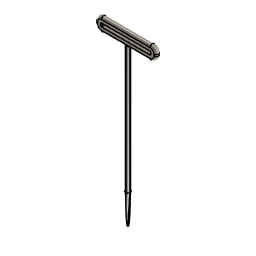
foamBrickElement (Autodesk Fusion 360 archive; units mm, degrees)
design "泡沫板_钉子"
Autodesk Fusion 360 part; units mm, degrees
sketch "草图1" plane through (0, 0, 0) normal (0, 1, 0) x (1, 0, 0)
  line L0 (0, 0) -> (0, -25.7)
  line L1 (0, -25.7) -> (-4.625, -25.7)
  line L2 (-4.625, -25.7) -> (-4.625, -28)
  line L3 (-4.625, -28) -> (5.375, -28)
  line L4 (5.375, -28) -> (5.375, -25.7)
  line L5 (5.375, -25.7) -> (0.75, -25.7)
  line L6 (0.75, -25.7) -> (0.75, 0)
  line L7 (0.75, 0) -> (0, 0)
  line L8 (0.375, -28) -> (0.375, 0)
  line L9 (0.375, 0) -> (0.375, -0.4348)
  line L10 (0.375, 0) -> (0.75, -5)
  line L11 (0.375, 0) -> (0, -5)
  line L12 (0.75, -5) -> (0, -5)
  dimension "d1" = 2.3
  dimension "d2" = 0.75
  dimension "d3" = 5
  dimension "d4" = 28
  dimension "d5" = 10
  constraint coincident L0.start L7.end
  constraint vertical L0
  constraint perpendicular L0 L1
  constraint perpendicular L1 L2
  constraint perpendicular L2 L3
  constraint perpendicular L2 L5
  constraint perpendicular L1 L6
  constraint perpendicular L0 L7
  constraint perpendicular L4 L5
  constraint midpoint L3 L8.start
  constraint midpoint L7 L8.end
  constraint perpendicular L3 L8
  constraint collinear L1 L5
  constraint coincident L8 L9.end
  constraint coincident L6 L10.end
  constraint coincident L0 L11.end
  constraint perpendicular L6 L12
  measures "d1" distance of L3.end L4.end
  measures "d2" distance of L0 L6
  measures "d3" distance of L7 L10.end
  measures "d4" distance of L3 L8.end
  measures "d5" distance of L2 L4
extrude "拉伸1" add sketch "草图1" along normal blind 0.75 contours L0 L1 L2 L3 L8 L12 | L8 L9 L11 L12 | L8 L9 L10 L12 | L3 L4 L5 L6 L8 L12
fillet "圆角1" radius 1 4 edges at (5.375, 0.375, 28) (5.375, 0.375, 25.7) (-4.625, 0.375, 25.7) (-4.625, 0.375, 28)
fillet "圆角2" radius 0.375 18 edges at (-1.8125, 0, 25.7) (-4.3321, 0, 25.9929) (-4.625, 0, 26.85) (-4.3321, 0, 27.7071) (0.375, 0, 28) (5.0821, 0, 27.7071) (5.375, 0, 26.85) (5.0821, 0, 25.9929) (2.5625, 0, 25.7) (-1.8125, 0.75, 25.7) (-4.3321, 0.75, 25.9929) (-4.625, 0.75, 26.85) (-4.3321, 0.75, 27.7071) (0.375, 0.75, 28) (5.0821, 0.75, 27.7071) (5.375, 0.75, 26.85) (5.0821, 0.75, 25.9929) (2.5625, 0.75, 25.7)
fillet "圆角3" radius 0.325 8 edges at (0.75, 0, 15.5375) (0.75, 0.75, 15.5375) (0, 0.75, 15.5375) (0, 0, 15.5375) (0.5625, 0, 2.5) (0.5625, 0.75, 2.5) (0.1875, 0, 2.5) (0.1875, 0.75, 2.5)
sketch "草图2" plane through (0, 0, 0) normal (0, -1, 0) x (1, 0, 0)
  line L0 (0.425, 26.075) -> (4.375, 26.075)
  arc A0 (4.375, 26.075) -> (5, 26.7) centre (4.375, 26.7) ccw
  line L1 (5, 26.7) -> (5, 27)
  arc A1 (5, 27) -> (4.375, 27.625) centre (4.375, 27) ccw
  line L2 (4.375, 27.625) -> (-3.625, 27.625)
  arc A2 (-3.625, 27.625) -> (-4.25, 27) centre (-3.625, 27) ccw
  line L3 (-4.25, 27) -> (-4.25, 26.7)
  arc A3 (-4.25, 26.7) -> (-3.625, 26.075) centre (-3.625, 26.7) ccw
  line L4 (-3.625, 26.075) -> (0.325, 26.075)
  line L5 (0.325, 26.075) -> (0.325, 5.0122)
  line L6 (0.325, 5.0122) -> (0.375, 4.3455)
  line L7 (0.375, 4.3455) -> (0.425, 5.0122)
  line L8 (0.425, 5.0122) -> (0.425, 26.075)
  line L9 (-3.75, 27) -> (-3.75, 26.7)
  arc A4 (-3.75, 26.7) -> (-3.625, 26.575) centre (-3.625, 26.7) ccw
  line L10 (-3.625, 26.575) -> (-0.075, 26.575)
  line L11 (-0.075, 26.575) -> (0.825, 26.575)
  line L12 (0.825, 26.575) -> (4.375, 26.575)
  arc A5 (4.375, 26.575) -> (4.5, 26.7) centre (4.375, 26.7) ccw
  line L13 (4.5, 26.7) -> (4.5, 27)
  arc A6 (4.5, 27) -> (4.375, 27.125) centre (4.375, 27) ccw
  line L14 (4.375, 27.125) -> (-3.625, 27.125)
  arc A7 (-3.625, 27.125) -> (-3.75, 27) centre (-3.625, 27) ccw
  dimension "d14" = -0.5
extrude "拉伸2" cut sketch "草图2" against normal blind 3 contours L9 A4 L10 L11 L12 A5 L13 A6 L14 A7
equation "d11 = ( 0.75 / 2 ) * 1 mm"

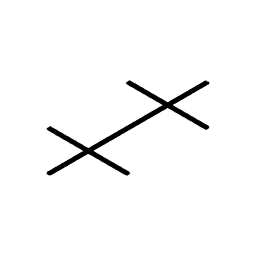
design "泡沫板_mark"
Autodesk Fusion 360 part; units mm, degrees
sketch "草图1" plane through (0, 0, 0) normal (0, 0, 1) x (1, 0, 0)
  line L0 (0, 0) -> (200, 0) construction
  line L1 (200, 0) -> (200, 400) construction
  line L2 (200, 400) -> (0, 400) construction
  line L3 (0, 400) -> (0, 0) construction
  line L4 (100, 400) -> (100, 0) construction
  line L5 (0, 300) -> (200, 300) construction
  line L6 (0, 100) -> (200, 100) construction
  line L7 (103.5, 0) -> (96.5, 0)
  line L8 (96.5, 0) -> (96.5, 400)
  line L9 (96.5, 400) -> (103.5, 400)
  line L10 (103.5, 400) -> (103.5, 0)
  line L11 (103.5, 0) -> (96.5, 400) construction
  line L12 (96.5, 0) -> (103.5, 400) construction
  line L13 (200, 96.5) -> (0, 96.5)
  line L14 (0, 96.5) -> (0, 103.5)
  line L15 (0, 103.5) -> (200, 103.5)
  line L16 (200, 103.5) -> (200, 96.5)
  line L17 (200, 96.5) -> (0, 103.5) construction
  line L18 (0, 96.5) -> (200, 103.5) construction
  line L19 (200, 296.5) -> (0, 296.5)
  line L20 (0, 296.5) -> (0, 303.5)
  line L21 (0, 303.5) -> (200, 303.5)
  line L22 (200, 303.5) -> (200, 296.5)
  line L23 (200, 296.5) -> (0, 303.5) construction
  line L24 (0, 296.5) -> (200, 303.5) construction
  point P0 (100, 200)
  point P1 (100, 100)
  point P2 (100, 300)
  dimension "d1" = 200
  dimension "d2" = 400
  dimension "d3" = 100
  dimension "d4" = 100
  dimension "d5" = 7
  dimension "d6" = 7
  dimension "d7" = 7
  constraint horizontal L0
  constraint vertical L1
  constraint horizontal L2
  constraint vertical L3
  constraint coincident L0.start L3.end
  constraint midpoint L2 L4.start
  constraint midpoint L0 L4.end
  constraint coincident L3 L5.start
  constraint coincident L1 L5.end
  constraint perpendicular L1 L5
  constraint coincident L3 L6.start
  constraint coincident L1 L6.end
  constraint perpendicular L1 L6
  constraint horizontal L7
  constraint perpendicular L7 L8
  constraint parallel L7 L9
  constraint parallel L8 L10
  constraint coincident L11 P0
  constraint coincident L12 P0
  constraint coincident L0 L7.start
  constraint midpoint L4 P0
  constraint horizontal L13
  constraint perpendicular L13 L14
  constraint parallel L13 L15
  constraint parallel L14 L16
  constraint coincident L17 P1
  constraint coincident L18 P1
  constraint coincident L1 L13.start
  constraint midpoint L6 P1
  constraint horizontal L19
  constraint perpendicular L19 L20
  constraint parallel L19 L21
  constraint parallel L20 L22
  constraint coincident L23 P2
  constraint coincident L24 P2
  constraint coincident L1 L19.start
  constraint midpoint L5 P2
  measures "d1" distance of L1.end L2.end
  measures "d2" distance of L0.end L1.end
  measures "d3" distance of L2 L5
  measures "d4" distance of L0 L6
  measures "d5" distance of L8 L10
  measures "d6" distance of L19 L21
  measures "d7" distance of L13 L15
extrude "拉伸1" add sketch "草图1" along normal blind 1 makes body 1
sketch "草图2" plane through (0, 0, 1) normal (0, 0, 1) x (-1, 0, 0)
  line L0 (-200, -303.5) -> (-103.5, -303.5)
  line L1 (-103.5, -303.5) -> (-103.5, -400)
  line L2 (-103.5, -400) -> (-96.5, -400)
  line L3 (-96.5, -400) -> (-96.5, -303.5)
  line L4 (-96.5, -303.5) -> (0, -303.5)
  line L5 (0, -303.5) -> (0, -296.5)
  line L6 (0, -296.5) -> (-96.5, -296.5)
  line L7 (-96.5, -296.5) -> (-96.5, -103.5)
  line L8 (-96.5, -103.5) -> (0, -103.5)
  line L9 (0, -103.5) -> (0, -96.5)
  line L10 (0, -96.5) -> (-96.5, -96.5)
  line L11 (-96.5, -96.5) -> (-96.5, 0)
  line L12 (-96.5, 0) -> (-103.5, 0)
  line L13 (-103.5, 0) -> (-103.5, -96.5)
  line L14 (-103.5, -96.5) -> (-200, -96.5)
  line L15 (-200, -96.5) -> (-200, -103.5)
  line L16 (-200, -103.5) -> (-103.5, -103.5)
  line L17 (-103.5, -103.5) -> (-103.5, -296.5)
  line L18 (-103.5, -296.5) -> (-200, -296.5)
  line L19 (-200, -296.5) -> (-200, -303.5)
  circle A0 centre (-100, -100) radius 2.5
  circle A1 centre (-199.994, -100) radius 2.5
  circle A2 centre (-194.112, -100) radius 2.5
  circle A3 centre (-188.23, -100) radius 2.5
  circle A4 centre (-182.348, -100) radius 2.5
  circle A5 centre (-176.466, -100) radius 2.5
  circle A6 centre (-170.584, -100) radius 2.5
  circle A7 centre (-164.702, -100) radius 2.5
  circle A8 centre (-158.82, -100) radius 2.5
  circle A9 centre (-152.938, -100) radius 2.5
  circle A10 centre (-147.056, -100) radius 2.5
  circle A11 centre (-141.174, -100) radius 2.5
  circle A12 centre (-135.292, -100) radius 2.5
  circle A13 centre (-129.41, -100) radius 2.5
  circle A14 centre (-123.528, -100) radius 2.5
  circle A15 centre (-117.646, -100) radius 2.5
  circle A16 centre (-111.764, -100) radius 2.5
  circle A17 centre (-105.882, -100) radius 2.5
  circle A18 centre (-94.118, -100) radius 2.5
  circle A19 centre (-88.236, -100) radius 2.5
  circle A20 centre (-82.354, -100) radius 2.5
  circle A21 centre (-76.472, -100) radius 2.5
  circle A22 centre (-70.59, -100) radius 2.5
  circle A23 centre (-64.708, -100) radius 2.5
  circle A24 centre (-58.826, -100) radius 2.5
  circle A25 centre (-52.944, -100) radius 2.5
  circle A26 centre (-47.062, -100) radius 2.5
  circle A27 centre (-41.18, -100) radius 2.5
  circle A28 centre (-35.298, -100) radius 2.5
  circle A29 centre (-29.416, -100) radius 2.5
  circle A30 centre (-23.534, -100) radius 2.5
  circle A31 centre (-17.652, -100) radius 2.5
  circle A32 centre (-11.77, -100) radius 2.5
  circle A33 centre (-100, -105.8824) radius 2.5
  circle A34 centre (-100, -111.7647) radius 2.5
  circle A35 centre (-100, -117.6471) radius 2.5
  circle A36 centre (-100, -123.5294) radius 2.5
  circle A37 centre (-100, -129.4118) radius 2.5
  circle A38 centre (-100, -135.2941) radius 2.5
  circle A39 centre (-100, -141.1765) radius 2.5
  circle A40 centre (-100, -147.0588) radius 2.5
  circle A41 centre (-100, -152.9412) radius 2.5
  circle A42 centre (-100, -158.8235) radius 2.5
  circle A43 centre (-100, -164.7059) radius 2.5
  circle A44 centre (-100, -170.5882) radius 2.5
  circle A45 centre (-100, -176.4706) radius 2.5
  circle A46 centre (-100, -182.3529) radius 2.5
  circle A47 centre (-100, -188.2353) radius 2.5
  circle A48 centre (-100, -194.1176) radius 2.5
  circle A49 centre (-100, -200) radius 2.5
  circle A50 centre (-100, -205.8824) radius 2.5
  circle A51 centre (-100, -211.7647) radius 2.5
  circle A52 centre (-100, -217.6471) radius 2.5
  circle A53 centre (-100, -223.5294) radius 2.5
  circle A54 centre (-100, -229.4118) radius 2.5
  circle A55 centre (-100, -235.2941) radius 2.5
  circle A56 centre (-100, -241.1765) radius 2.5
  circle A57 centre (-100, -247.0588) radius 2.5
  circle A58 centre (-100, -252.9412) radius 2.5
  circle A59 centre (-100, -258.8235) radius 2.5
  circle A60 centre (-100, -264.7059) radius 2.5
  circle A61 centre (-100, -270.5882) radius 2.5
  circle A62 centre (-100, -276.4706) radius 2.5
  circle A63 centre (-100, -282.3529) radius 2.5
  circle A64 centre (-100, -288.2353) radius 2.5
  circle A65 centre (-100, -294.1176) radius 2.5
  circle A66 centre (-100, -300) radius 2.5
  circle A67 centre (-5.888, -100) radius 2.5
  circle A68 centre (-0.006, -100) radius 2.5
  circle A69 centre (-100, -94.118) radius 2.5
  circle A70 centre (-100, -88.236) radius 2.5
  circle A71 centre (-100, -82.354) radius 2.5
  circle A72 centre (-100, -76.472) radius 2.5
  circle A73 centre (-100, -70.59) radius 2.5
  circle A74 centre (-100, -64.708) radius 2.5
  circle A75 centre (-100, -58.826) radius 2.5
  circle A76 centre (-100, -52.944) radius 2.5
  circle A77 centre (-100, -47.062) radius 2.5
  circle A78 centre (-100, -41.18) radius 2.5
  circle A79 centre (-100, -35.298) radius 2.5
  circle A80 centre (-100, -29.416) radius 2.5
  circle A81 centre (-100, -23.534) radius 2.5
  circle A82 centre (-100, -17.652) radius 2.5
  circle A83 centre (-100, -11.77) radius 2.5
  circle A84 centre (-100, -5.888) radius 2.5
  circle A85 centre (-100, -0.006) radius 2.5
  circle A86 centre (-100, -305.882) radius 2.5
  circle A87 centre (-100, -311.764) radius 2.5
  circle A88 centre (-100, -317.646) radius 2.5
  circle A89 centre (-100, -323.528) radius 2.5
  circle A90 centre (-100, -329.41) radius 2.5
  circle A91 centre (-100, -335.292) radius 2.5
  circle A92 centre (-100, -341.174) radius 2.5
  circle A93 centre (-100, -347.056) radius 2.5
  circle A94 centre (-100, -352.938) radius 2.5
  circle A95 centre (-100, -358.82) radius 2.5
  circle A96 centre (-100, -364.702) radius 2.5
  circle A97 centre (-100, -370.584) radius 2.5
  circle A98 centre (-100, -376.466) radius 2.5
  circle A99 centre (-100, -382.348) radius 2.5
  circle A100 centre (-100, -388.23) radius 2.5
  circle A101 centre (-100, -394.112) radius 2.5
  circle A102 centre (-100, -399.994) radius 2.5
  circle A103 centre (-199.994, -300) radius 2.5
  circle A104 centre (-194.112, -300) radius 2.5
  circle A105 centre (-188.23, -300) radius 2.5
  circle A106 centre (-182.348, -300) radius 2.5
  circle A107 centre (-176.466, -300) radius 2.5
  circle A108 centre (-170.584, -300) radius 2.5
  circle A109 centre (-164.702, -300) radius 2.5
  circle A110 centre (-158.82, -300) radius 2.5
  circle A111 centre (-152.938, -300) radius 2.5
  circle A112 centre (-147.056, -300) radius 2.5
  circle A113 centre (-141.174, -300) radius 2.5
  circle A114 centre (-135.292, -300) radius 2.5
  circle A115 centre (-129.41, -300) radius 2.5
  circle A116 centre (-123.528, -300) radius 2.5
  circle A117 centre (-117.646, -300) radius 2.5
  circle A118 centre (-111.764, -300) radius 2.5
  circle A119 centre (-105.882, -300) radius 2.5
  circle A120 centre (-94.118, -300) radius 2.5
  circle A121 centre (-88.236, -300) radius 2.5
  circle A122 centre (-82.354, -300) radius 2.5
  circle A123 centre (-76.472, -300) radius 2.5
  circle A124 centre (-70.59, -300) radius 2.5
  circle A125 centre (-64.708, -300) radius 2.5
  circle A126 centre (-58.826, -300) radius 2.5
  circle A127 centre (-52.944, -300) radius 2.5
  circle A128 centre (-47.062, -300) radius 2.5
  circle A129 centre (-41.18, -300) radius 2.5
  circle A130 centre (-35.298, -300) radius 2.5
  circle A131 centre (-29.416, -300) radius 2.5
  circle A132 centre (-23.534, -300) radius 2.5
  circle A133 centre (-17.652, -300) radius 2.5
  circle A134 centre (-11.77, -300) radius 2.5
  circle A135 centre (-5.888, -300) radius 2.5
  circle A136 centre (-0.006, -300) radius 2.5
  dimension "d10" = 5
  dimension "d11" = 3.5
  dimension "d12" = 3.5
  dimension "d15" = 5.882
  dimension "d16" = 0
  dimension "d19" = 0
  dimension "d20" = -200
  dimension "d23" = 0
  dimension "d24" = 5.882
  dimension "d27" = 0
  dimension "d28" = -5.882
  dimension "d31" = 5.882
  dimension "d32" = 0
  measures "d10" diameter of A0
  measures "d11" distance of L14 A0.centre
  measures "d12" distance of L17 A0.centre
extrude "拉伸2" add sketch "草图2" along normal blind 1 contours L0 L1 L2 L3 L4 L5 L6 L7 L8 L9 L10 L11 L12 L13 L14 L15 L16 L17 L18 L19 A1 A68 A85 A102 A103 A136 bodies 1
extrude "拉伸1'" add 137 faces at (99.3115, 252.2233, 1) (98.3961, 330.0884, 1) (198.6178, 99.2032, 1) (115.8857, 100.1944, 1) (148.0377, 100.5668, 1) (100.3045, 263.9302, 1) (100.3045, 287.4596, 1) (42.867, 99.7086, 1) (21.6072, 99.6697, 1) (100.3045, 275.6949, 1) (54.631, 99.7086, 1) (11.4614, 100.831, 1) (195.0937, 100.5668, 1) (100.3045, 363.9263, 1) (99.3115, 246.341, 1) (98.3961, 341.8524, 1) (86.4757, 100.1944, 1) (98.3961, 318.3244, 1) (60.513, 99.7086, 1) (100.3045, 334.5163, 1) (100.3045, 281.5772, 1) (99.3115, 222.8116, 1) (99.3115, 216.9292, 1) (136.2737, 100.5668, 1) (66.4683, 100.1944, 1) (72.3503, 100.1944, 1) (48.749, 99.7086, 1) (110.0037, 100.1944, 1) (130.3917, 100.5668, 1) (99.3115, 234.5763, 1) (142.1557, 100.5668, 1) (98.3961, 271.2666, 1) (153.9197, 100.5668, 1) (165.6837, 100.5668, 1) (36.985, 99.7086, 1) (107.6423, 100.1944, 1) (159.8017, 100.5668, 1) (80.5937, 100.1944, 1) (5.5794, 100.831, 1) (121.7677, 100.1944, 1) (95.8783, 100.1944, 1) (171.5657, 100.5668, 1) (177.4477, 100.5668, 1) (99.3115, 211.0469, 1) (183.3297, 100.5668, 1) (0.7165, 99.2742, 1) (189.2117, 100.5668, 1) (100.5196, 59.7259, 1) (53.2485, 299.2243, 1) (101.7603, 106.0767, 1) (101.7603, 70.7844, 1) (99.3115, 134.5763, 1) (100.5196, 53.8439, 1) (59.1305, 299.2243, 1) (99.3115, 199.2822, 1) (117.9505, 299.2243, 1) (99.3115, 163.988, 1) (99.3115, 158.1057, 1) (101.7603, 88.4304, 1) (99.6955, 12.5457, 1) (100.5196, 47.9619, 1) (99.3115, 169.8704, 1) (135.5965, 299.2243, 1) (101.7603, 94.3124, 1) (188.5345, 299.2243, 1) (100.6983, 0.5948, 1) (101.7603, 76.6664, 1) (99.3115, 175.7528, 1) (100.0623, 131.1816, 1) (99.3115, 28.6982, 1) (100.3045, 299.2243, 1) (94.4225, 299.2243, 1) (170.8885, 299.2243, 1) (199.167, 300.0624, 1) (99.3115, 181.6351, 1) (176.7705, 299.2243, 1) (17.3475, 299.2243, 1) (101.7603, 100.1944, 1) (99.6955, 6.6637, 1) (100.5196, 42.0799, 1) (0.833, 300.0624, 1) (101.7603, 117.8414, 1) (99.5601, 19.0214, 1) (88.5405, 299.2243, 1) (6.1925, 299.2243, 1) (101.7603, 123.7238, 1) (82.6585, 299.2243, 1) (112.0685, 299.2243, 1) (70.8945, 299.2243, 1) (100.5196, 36.1979, 1) (99.3115, 152.2233, 1) (194.4165, 299.2243, 1) (99.3115, 146.341, 1) (99.3115, 187.5175, 1) (101.7603, 111.9591, 1) (106.1865, 299.2243, 1) (123.8325, 299.2243, 1) (99.3115, 193.3998, 1) (182.6525, 299.2243, 1) (99.3115, 22.8162, 1) (147.3605, 299.2243, 1) (101.7603, 82.5484, 1) (99.3115, 140.4586, 1) (65.0125, 299.2243, 1) (12.0745, 299.2243, 1) (76.7765, 299.2243, 1) (99.4602, 65.4483, 1) (35.6025, 299.2243, 1) (27.4892, 99.6697, 1) (23.2295, 299.2243, 1) (41.4845, 299.2243, 1) (165.0065, 299.2243, 1) (141.4785, 299.2243, 1) (74.7117, 100.1944, 1) (100.3045, 293.3419, 1) (159.1245, 299.2243, 1) (129.7145, 299.2243, 1) (29.1115, 299.2243, 1) (47.3665, 299.2243, 1) (153.2425, 299.2243, 1) (17.7129, 100.8124, 1) (100.3045, 352.1623, 1) (100.3045, 310.9883, 1) (98.3961, 306.5604, 1) (100.3045, 322.7523, 1) (99.3115, 240.4586, 1) (98.3961, 259.5019, 1) (98.3961, 371.2624, 1) (99.3115, 205.1645, 1) (98.3961, 394.7904, 1) (98.3961, 359.4984, 1) (99.3115, 228.6939, 1) (99.6281, 398.6683, 1) (100.3045, 387.4543, 1) (98.3961, 383.0264, 1) (100.3045, 375.6903, 1) (98.3961, 347.7344, 1) along direction (0, 0, 1) blind 1 separate body on bodies 1 makes body 2 at (100.3045, 375.6903, 1) makes body 3 at (100.3045, 387.4543, 1) makes body 4 at (99.3115, 228.6939, 1) makes body 5 at (98.3961, 394.7904, 1) makes body 6 at (98.3961, 371.2624, 1) makes body 7 at (99.3115, 240.4586, 1) makes body 8 at (98.3961, 306.5604, 1) makes body 9 at (100.3045, 352.1623, 1) makes body 10 at (153.2425, 299.2243, 1) makes body 11 at (29.1115, 299.2243, 1) makes body 12 at (159.1245, 299.2243, 1) makes body 13 at (74.7117, 100.1944, 1) makes body 14 at (165.0065, 299.2243, 1) makes body 15 at (23.2295, 299.2243, 1) makes body 16 at (35.6025, 299.2243, 1) makes body 17 at (76.7765, 299.2243, 1) makes body 18 at (65.0125, 299.2243, 1) makes body 19 at (101.7603, 82.5484, 1) makes body 20 at (99.3115, 22.8162, 1) makes body 21 at (99.3115, 193.3998, 1) makes body 22 at (106.1865, 299.2243, 1) makes body 23 at (99.3115, 187.5175, 1) makes body 24 at (194.4165, 299.2243, 1) makes body 25 at (100.5196, 36.1979, 1) makes body 26 at (112.0685, 299.2243, 1) makes body 27 at (101.7603, 123.7238, 1) makes body 28 at (88.5405, 299.2243, 1) makes body 29 at (101.7603, 117.8414, 1) makes body 30 at (100.5196, 42.0799, 1) makes body 31 at (101.7603, 100.1944, 1) makes body 32 at (176.7705, 299.2243, 1) makes body 33 at (199.167, 300.0624, 1) makes body 34 at (94.4225, 299.2243, 1) makes body 35 at (99.3115, 28.6982, 1) makes body 36 at (99.3115, 175.7528, 1) makes body 37 at (100.6983, 0.5948, 1) makes body 38 at (101.7603, 94.3124, 1) makes body 39 at (99.3115, 169.8704, 1) makes body 40 at (99.6955, 12.5457, 1) makes body 41 at (99.3115, 158.1057, 1) makes body 42 at (117.9505, 299.2243, 1) makes body 43 at (59.1305, 299.2243, 1) makes body 44 at (99.3115, 134.5763, 1) makes body 45 at (101.7603, 106.0767, 1) makes body 46 at (100.5196, 59.7259, 1) makes body 47 at (0.7165, 99.2742, 1) makes body 48 at (99.3115, 211.0469, 1) makes body 49 at (171.5657, 100.5668, 1) makes body 50 at (121.7677, 100.1944, 1) makes body 51 at (80.5937, 100.1944, 1) makes body 52 at (107.6423, 100.1944, 1) makes body 53 at (165.6837, 100.5668, 1) makes body 54 at (98.3961, 271.2666, 1) makes body 55 at (99.3115, 234.5763, 1) makes body 56 at (110.0037, 100.1944, 1) makes body 57 at (72.3503, 100.1944, 1) makes body 58 at (136.2737, 100.5668, 1) makes body 59 at (99.3115, 222.8116, 1) makes body 60 at (100.3045, 334.5163, 1) makes body 61 at (98.3961, 318.3244, 1) makes body 62 at (98.3961, 341.8524, 1) makes body 63 at (100.3045, 363.9263, 1) makes body 64 at (11.4614, 100.831, 1) makes body 65 at (100.3045, 275.6949, 1) makes body 66 at (42.867, 99.7086, 1) makes body 67 at (100.3045, 263.9302, 1) makes body 68 at (115.8857, 100.1944, 1) makes body 69 at (98.3961, 330.0884, 1) makes body 70 at (99.3115, 252.2233, 1) makes body 71 at (198.6178, 99.2032, 1) makes body 72 at (148.0377, 100.5668, 1) makes body 73 at (100.3045, 287.4596, 1) makes body 74 at (21.6072, 99.6697, 1) makes body 75 at (54.631, 99.7086, 1) makes body 76 at (195.0937, 100.5668, 1) makes body 77 at (99.3115, 246.341, 1) makes body 78 at (86.4757, 100.1944, 1) makes body 79 at (60.513, 99.7086, 1) makes body 80 at (100.3045, 281.5772, 1) makes body 81 at (99.3115, 216.9292, 1) makes body 82 at (66.4683, 100.1944, 1) makes body 83 at (48.749, 99.7086, 1) makes body 84 at (130.3917, 100.5668, 1) makes body 85 at (142.1557, 100.5668, 1) makes body 86 at (153.9197, 100.5668, 1) makes body 87 at (36.985, 99.7086, 1) makes body 88 at (159.8017, 100.5668, 1) makes body 89 at (5.5794, 100.831, 1) makes body 90 at (95.8783, 100.1944, 1) makes body 91 at (177.4477, 100.5668, 1) makes body 92 at (183.3297, 100.5668, 1) makes body 93 at (189.2117, 100.5668, 1) makes body 94 at (53.2485, 299.2243, 1) makes body 95 at (101.7603, 70.7844, 1) makes body 96 at (100.5196, 53.8439, 1) makes body 97 at (99.3115, 199.2822, 1) makes body 98 at (99.3115, 163.988, 1) makes body 99 at (101.7603, 88.4304, 1) makes body 100 at (100.5196, 47.9619, 1) makes body 101 at (135.5965, 299.2243, 1) makes body 102 at (188.5345, 299.2243, 1) makes body 103 at (101.7603, 76.6664, 1) makes body 104 at (100.0623, 131.1816, 1) makes body 105 at (100.3045, 299.2243, 1) makes body 106 at (170.8885, 299.2243, 1) makes body 107 at (99.3115, 181.6351, 1) makes body 108 at (17.3475, 299.2243, 1) makes body 109 at (99.6955, 6.6637, 1) makes body 110 at (0.833, 300.0624, 1) makes body 111 at (99.5601, 19.0214, 1) makes body 112 at (6.1925, 299.2243, 1) makes body 113 at (82.6585, 299.2243, 1) makes body 114 at (70.8945, 299.2243, 1) makes body 115 at (99.3115, 152.2233, 1) makes body 116 at (99.3115, 146.341, 1) makes body 117 at (101.7603, 111.9591, 1) makes body 118 at (123.8325, 299.2243, 1) makes body 119 at (182.6525, 299.2243, 1) makes body 120 at (147.3605, 299.2243, 1) makes body 121 at (99.3115, 140.4586, 1) makes body 122 at (12.0745, 299.2243, 1) makes body 123 at (99.4602, 65.4483, 1) makes body 124 at (27.4892, 99.6697, 1) makes body 125 at (41.4845, 299.2243, 1) makes body 126 at (141.4785, 299.2243, 1) makes body 127 at (100.3045, 293.3419, 1) makes body 128 at (129.7145, 299.2243, 1) makes body 129 at (47.3665, 299.2243, 1) makes body 130 at (17.7129, 100.8124, 1) makes body 131 at (100.3045, 310.9883, 1) makes body 132 at (100.3045, 322.7523, 1) makes body 133 at (98.3961, 259.5019, 1) makes body 134 at (99.3115, 205.1645, 1) makes body 135 at (98.3961, 359.4984, 1) makes body 136 at (99.6281, 398.6683, 1) makes body 137 at (98.3961, 383.0264, 1) makes body 138 at (98.3961, 347.7344, 1) in component "Component'"
component "Component'" placed x (1, 0, 0) y (0, 1, 0) z (0, 0, 1) at (0, 0, 0)
